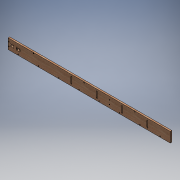
# Autodesk Inventor part: licht_200_top_a
Saved by Autodesk Inventor 2016 SP2 (Build 200236200, 236)
## iProperties
Created: 2018-01-11
Part Number: licht_200_top_a
Material: Spanplatte
Document SubType Name: Blech
Designer: schueler
Density: 1 g/cm^3
Sheet Metal Rule: Standard_mm
Appearance: Birke - natur- poliert
Mass: 2499.25 g
Surface Area: 3823.01 cm^2
Volume: 2499.25 cm^3
Author: schueler
Autodesk Inventor part; units mm, degrees
ref_plane "YZ Plane" through (0, 0, 0) normal (1, 0, 0) x (0, 1, 0)
ref_plane "XZ Plane" through (0, 0, 0) normal (0, 1, 0) x (-1, 0, 0)
ref_plane "XY Plane" through (0, 0, 0) normal (0, 0, 1) x (1, 0, 0)
sketch "Skizze1" plane through (0, 0, 0) normal (0, 1, 0) x (-1, 0, 0)
  line L0 (0, 0) -> (1600, 0)
  line L1 (1600, 0) -> (1600, -100)
  line L2 (1600, -100) -> (0, -100)
  line L3 (475, 0) -> (475, -100) construction
  line L4 (725, 0) -> (725, -100) construction
  line L5 (1500, 0) -> (1500, -100) construction
  line L6 (0, -92) -> (1600, -92) construction
  circle A0 centre (1500, -92) radius 1.5
  line L7 (1592, 0) -> (1592, -100) construction
  circle A1 centre (1592, -70) radius 1.5
  circle A2 centre (1592, -30) radius 1.5
  line L8 (975, -137) -> (975, -21) construction
  line L9 (1600, -8) -> (0, -8) construction
  circle A3 centre (1350, -8) radius 1.5
  line L10 (100, 0) -> (100, -100) construction
  line L11 (225, 0) -> (225, -100) construction
  line L12 (1300, 0) -> (1300, -100) construction
  line L13 (1100, 0) -> (1100, -100) construction
  line L14 (900, 0) -> (900, -100) construction
  line L15 (225, -16) -> (225, -16)
  line L16 (220, -21) -> (220, -79)
  line L17 (225, -84) -> (225, -84)
  line L18 (230, -79) -> (230, -21)
  arc A4 (230, -21) -> (225, -16) centre (225, -21) ccw
  arc A5 (225, -16) -> (220, -21) centre (225, -21) ccw
  arc A6 (220, -79) -> (225, -84) centre (225, -79) ccw
  arc A7 (225, -84) -> (230, -79) centre (225, -79) ccw
  circle A8 centre (100, -92) radius 1.5
  circle A9 centre (1300, -92) radius 1.5
  circle A10 centre (1100, -92) radius 1.5
  line L19 (300, 0) -> (300, -100) construction
  circle A11 centre (350, -8) radius 1.5
  circle A12 centre (300, -92) radius 1.5
  circle A13 centre (900, -92) radius 1.5
  circle A14 centre (850, -8) radius 1.5
  line L20 (500, 0) -> (500, -100) construction
  line L21 (700, 0) -> (700, -100) construction
  circle A15 centre (500, -92) radius 1.5
  circle A16 centre (700, -92) radius 1.5
  line L22 (475, -16) -> (475, -16)
  line L23 (470, -21) -> (470, -79)
  line L24 (480, -79) -> (480, -21)
  line L25 (975, -84) -> (225, -84) construction
  line L26 (225, -16) -> (975, -16) construction
  line L27 (975, -21) -> (225, -21) construction
  line L28 (225, -79) -> (975, -79) construction
  line L29 (725, -16) -> (725, -16)
  line L30 (720, -21) -> (720, -79)
  line L31 (725, -84) -> (725, -84)
  line L32 (730, -79) -> (730, -21)
  line L33 (975, -16) -> (975, -16)
  line L34 (980, -21) -> (980, -79)
  line L35 (975, -84) -> (975, -84)
  line L36 (970, -79) -> (970, -21)
  arc A17 (980, -21) -> (975, -16) centre (975, -21) ccw
  arc A18 (975, -16) -> (970, -21) centre (975, -21) ccw
  arc A19 (970, -79) -> (975, -84) centre (975, -79) ccw
  arc A20 (975, -84) -> (980, -79) centre (975, -79) ccw
  arc A21 (720, -79) -> (725, -84) centre (725, -79) ccw
  arc A22 (725, -84) -> (730, -79) centre (725, -79) ccw
  arc A23 (730, -21) -> (725, -16) centre (725, -21) ccw
  arc A24 (725, -16) -> (720, -21) centre (725, -21) ccw
  arc A25 (480, -21) -> (475, -16) centre (475, -21) ccw
  arc A26 (475, -16) -> (470, -21) centre (475, -21) ccw
  arc A27 (470, -79) -> (475, -84) centre (475, -79) ccw
  arc A28 (475, -84) -> (480, -79) centre (475, -79) ccw
  line L37 (0, -100) -> (0, 0)
  point P0 (1500, -8)
  point P1 (225, -16)
  point P2 (300, -8)
  point P3 (900, -8)
  point P4 (480, -16)
  point P5 (470, -84)
  point P6 (470, -16)
  point P7 (480, -84)
  point P8 (475, -16)
  point P9 (730, -16)
  point P10 (720, -84)
  point P11 (720, -16)
  point P12 (730, -84)
  point P13 (970, -16)
  point P14 (980, -84)
  point P15 (980, -16)
  point P16 (970, -84)
  dimension "d2" = 1600
  dimension "d3" = 100
  dimension "d8" = 100
  dimension "d15" = 8
  dimension "d18" = 3
  dimension "d20" = 8
  dimension "d25" = 3
  dimension "d26" = 3
  dimension "d44" = 30
  dimension "d45" = 30
  dimension "d50" = 250
  dimension "d59" = 3
  dimension "d60" = 200
  dimension "d61" = 200
  dimension "d62" = 200
  dimension "d66" = 10
  dimension "d67" = 5
  dimension "d70" = 3
  dimension "d72" = 3
  dimension "d74" = 3
  dimension "d78" = 250
  dimension "d79" = 200
  dimension "d80" = 3
  dimension "d81" = 3
  dimension "d82" = 3
  dimension "d83" = 3
  dimension "d92" = 200
  dimension "d93" = 200
  dimension "d95" = 3
  dimension "d96" = 3
  dimension "d102" = 10
  dimension "d103" = 16
  dimension "d104" = 16
  dimension "d107" = 10
  dimension "d108" = 10
  dimension "d111" = 5
  dimension "d112" = 5
  dimension "d113" = 5
  dimension "d114" = 250
  dimension "d115" = 500
  dimension "d120" = 8
  dimension "d121" = 100
  dimension "d122" = 250
  dimension "d123" = 875
  dimension "d124" = 350
  constraints: 70 end point, 55 point on line, 32 point on circle, 31 tangent, 29 centre point, 15 vertical, 12 equal radius, 9 parallel, 6 horizontal, 5 midpoint, 5 perpendicular, 1 collinear, 48 other
  measures "d2" distance of L1.end L37.start
  measures "d3" distance of L1.start L1.end
  measures "d8" distance of L1.start L5.start
  measures "d15" distance of L37.start point (0, -92)
  measures "d18" diameter of A0
  measures "d20" distance of L1.start L7.start
  measures "d25" diameter of A1
  measures "d26" diameter of A2
  measures "d50" distance between parallel lines of L4 L8
  measures "d59" diameter of A3
  measures "d60" distance between parallel lines of L12 L5
  measures "d61" distance between parallel lines of L13 L12
  measures "d62" distance between parallel lines of L14 L13
  measures "d66" distance between parallel lines of L16 L18
  measures "d67" radius of A4
  measures "d70" diameter of A8
  measures "d72" diameter of A9
  measures "d74" diameter of A10
  measures "d78" distance between parallel lines of L3 L11
  measures "d79" distance between parallel lines of L10 L19
  measures "d80" diameter of A11
  measures "d81" diameter of A12
  measures "d82" diameter of A13
  measures "d83" diameter of A14
  measures "d92" distance between parallel lines of L19 L20
  measures "d93" distance between parallel lines of L14 L21
  measures "d95" diameter of A15
  measures "d96" diameter of A16
  measures "d102" distance between parallel lines of L23 L24
  measures "d103" distance of the line from the sketch origin of L26
  measures "d107" distance between parallel lines of L36 L34
  measures "d108" distance between parallel lines of L30 L32
  measures "d111" radius of A17
  measures "d112" radius of A21
  measures "d113" radius of A25
  measures "d114" distance from line of L1 A3.centre
  measures "d115" distance of A3.centre A14.centre
  measures "d120" distance of the line from the sketch origin of L9
  measures "d121" distance between parallel lines of L37 L10
  measures "d122" distance between parallel lines of L3 L4
  measures "d123" distance between parallel lines of L4 L1
  measures "d124" distance from line of L37 A11.centre
extrude "Extrusion9" add sketch "Skizze1" along normal blind 16
sketch "Skizze4" plane through (0, 0, 0) normal (0, -1, 0) x (1, 0, 0)
  circle A0 centre (-100, -92) radius 1.5 projected
  circle A1 centre (-300, -92) radius 1.5 projected
  circle A2 centre (-350, -8) radius 1.5 projected
  circle A3 centre (-500, -92) radius 1.5 projected
  circle A4 centre (-700, -92) radius 1.5 projected
  circle A5 centre (-850, -8) radius 1.5 projected
  circle A6 centre (-900, -92) radius 1.5 projected
  circle A7 centre (-1100, -92) radius 1.5 projected
  circle A8 centre (-1300, -92) radius 1.5 projected
  circle A9 centre (-1500, -92) radius 1.5 projected
  circle A10 centre (-1350, -8) radius 1.5 projected
  circle A11 centre (-1592, -30) radius 1.5 projected
  circle A12 centre (-1592, -70) radius 1.5 projected
  line L0 (-1600, -100) -> (0, -100) construction
  line L1 (0, -100) -> (0, 0) construction
  line L2 (0, 0) -> (-1600, 0) construction
  line L3 (-1600, 0) -> (-1600, -100) construction
  line L4 (-1600, 0) -> (0, 0) construction
  line L5 (-600, 0) -> (-600, -100) construction
  point P0 (-600, -30)
  point P1 (-600, -70)
  dimension "d132" = 1000
  dimension "d133" = 30
  dimension "d162" = 70
  constraints: 10 end point, 4 point on line, 2 parallel, 2 perpendicular, 1 horizontal
  measures "d132" distance between parallel lines of L3 L5
  measures "d133" distance of L5.start point (-600, -30)
  measures "d162" distance from line of point (-600, -70) L4
hole "Bohrung3" at (-850, 0, -8) at (-900, 0, -92) at (-700, 0, -92) at (-500, 0, -92) at (-350, 0, -8) at (-300, 0, -92) at (-100, 0, -92) at (-1100, 0, -92) at (-1300, 0, -92) at (-1350, 0, -8) at (-1500, 0, -92) at (-1592, 0, -70) at (-1592, 0, -30) at (-600, 0, -70) at (-600, 0, -30) direction (0, 1, 0) diameter 4 end through all countersink diameter 8 countersink angle 90
sketch "Skizze5" plane through (0, 0, 0) normal (0, -1, 0) x (1, 0, 0)
  line L0 (-1600, 0) -> (-1600, -100) construction
  line L1 (-1600, -50) -> (-1560, -50) construction
  line L2 (-1574.6, -35.4) -> (-1545.4, -35.4) construction
  line L3 (-1545.4, -35.4) -> (-1545.4, -64.6) construction
  line L4 (-1545.4, -64.6) -> (-1574.6, -64.6) construction
  line L5 (-1574.6, -64.6) -> (-1574.6, -35.4) construction
  line L6 (-1560, 0) -> (-1560, -100) construction
  line L7 (0, -100) -> (-1600, -100) construction
  circle A0 centre (-1560, -50) radius 25.4 construction
  line L8 (-1514.6, -35.4) -> (-1485.4, -35.4) construction
  line L9 (-1485.4, -35.4) -> (-1485.4, -64.6) construction
  line L10 (-1485.4, -64.6) -> (-1514.6, -64.6) construction
  line L11 (-1514.6, -64.6) -> (-1514.6, -35.4) construction
  line L12 (-1600, 0) -> (0, 0) construction
  line L13 (-1500, 0) -> (-1500, -100) construction
  circle A1 centre (-1500, -50) radius 25.4 construction
  point P0 (-1560, -35.4)
  point P1 (-1574.6, -50)
  point P2 (-1500, -35.4)
  dimension "d136" = 40
  dimension "d137" = 29.2
  dimension "d138" = 29.2
  dimension "d153" = 50.8
  dimension "d154" = 60
  dimension "d155" = 29.2
  dimension "d156" = 50.8
  dimension "d157" = 29.2
  constraints: 24 end point, 11 coincident, 6 midpoint, 6 point on line, 4 parallel, 3 horizontal, 3 perpendicular, 2 centre point, 2 vertical, 1 collinear
  measures "d136" distance between parallel lines of L0 L6
  measures "d137" distance of L3.end L4.end
  measures "d138" distance of L2.end L3.end
  measures "d153" diameter of A0
  measures "d154" distance between parallel lines of L13 L6
  measures "d155" distance of L8.start L8.end
  measures "d156" diameter of A1
  measures "d157" distance of L8.end L9.end
hole "Bohrung4" at (-1574.6, 0, -35.4) at (-1545.4, 0, -64.6) at (-1545.4, 0, -35.4) at (-1574.6, 0, -64.6) at (-1514.6, 0, -35.4) at (-1485.4, 0, -35.4) at (-1485.4, 0, -64.6) at (-1514.6, 0, -64.6) direction (0, 1, 0) diameter 1.5 end through all
hole "Bohrung5" at (-1560, 0, -50) at (-1500, 0, -50) direction (0, 1, 0) diameter 24 end through all
sketch "Skizze6" plane through (0, 0, 0) normal (0, -1, 0) x (1, 0, 0)
  circle A0 centre (-1500, -50) radius 12 projected
  line L0 (-1517.5, -42.5) -> (-1482.5, -42.5)
  line L1 (-1482.5, -42.5) -> (-1482.5, -57.5)
  line L2 (-1482.5, -57.5) -> (-1517.5, -57.5)
  line L3 (-1517.5, -57.5) -> (-1517.5, -42.5)
  line L4 (-1500, -50) -> (-1482.5, -50) construction
  line L5 (-1500, -50) -> (-1500, -42.5) construction
  point P0 (0, 0)
  dimension "d158" = 15
  dimension "d159" = 35
  constraints: 12 end point, 3 perpendicular, 2 midpoint, 2 parallel, 1 horizontal
  measures "d158" distance of L0.end L1.end
  measures "d159" distance of L0.start L0.end
extrude "Extrusion10" cut sketch "Skizze6" against normal blind 2 contours A0 L2 L0 | A0 L0 L1 L2 | A0 L2 L3 L0
equation "\"Biegeradius\" = Stärke"
equation "\"BreiteBiegungsfreistellung\" = Stärke"
equation "\"TiefeBiegungsfreistellung\" = 0.5 * Stärke"
equation "\"GrößeEckenfreistellung\" = 4 * Stärke"
equation "\"MinimalRest\" = 2 * Stärke"
equation "\"Übergangsradius\" = Biegeradius"
equation "\"JacobiRadiusGröße\" = Biegeradius"
equation "\"Abstandsgröße\" = Stärke"
equation "\"Stärke\" = 0.5"
